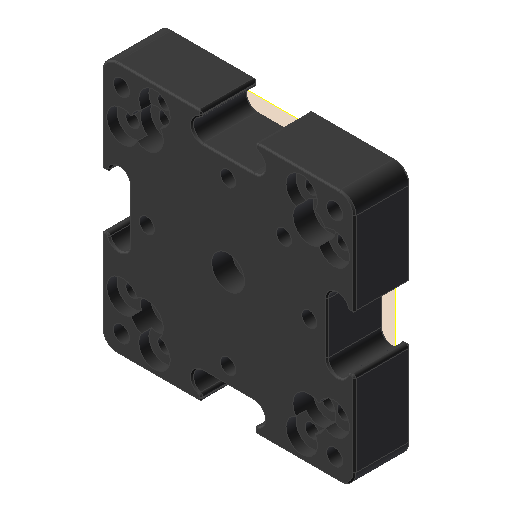
# Autodesk Inventor part: 40_XYZstage_micrometer_motorized_nema8_cube_ontop
Saved by Autodesk Inventor 2025.1 (Build 291241020, 241B)
## iProperties
Created: 2023-06-28
Part Number: 40_XYZstage_micrometer_motorized_nema8_cube_ontop
Material: Generisch
Document SubType Name: Modeling
Designer: diederichbenedict
Density: 1 g/cm^3
Appearance: Vorgabe
Author: diederichbenedict
Autodesk Inventor part; units mm, degrees
ref_plane "YZ Plane" through (0, 0, 0) normal (1, 0, 0) x (0, 1, 0)
ref_plane "XZ Plane" through (0, 0, 0) normal (0, 1, 0) x (-1, 0, 0)
ref_plane "XY Plane" through (0, 0, 0) normal (0, 0, 1) x (1, 0, 0)
ref_plane "Arbeitsebene1" through (0, 0, 0) normal (0, 0, 1) x (1, 0, 0)
sketch "Skizze1" plane through (0, 0, 0) normal (0, 0, 1) x (1, 0, 0)
  line L0 (0, -40) -> (0, 0) projected
  line L1 (0, 0) -> (-40, 0) projected
  line L2 (-40, 0) -> (-40, -40) projected
  line L3 (-40, -40) -> (0, -40) projected
  circle A0 centre (-20, -20) radius 1.5 projected
  circle A1 centre (-4, -20) radius 1.5 projected
  circle A2 centre (-4, -4) radius 1.5 projected
  circle A3 centre (-20, -4) radius 1.5 projected
  circle A4 centre (-36, -4) radius 1.5 projected
  circle A5 centre (-36, -20) radius 1.5 projected
  circle A6 centre (-36, -36) radius 1.5 projected
  circle A7 centre (-20, -36) radius 1.5 projected
  circle A8 centre (-4, -36) radius 1.5 projected
  circle A9 centre (-9, -8.5) radius 1.5 projected
  line L4 (1.9, 4.9) -> (-41.9, 4.9)
  line L5 (-44.9, 1.9) -> (-44.9, -41.9)
  line L6 (-41.9, -44.9) -> (1.9, -44.9)
  line L7 (4.9, -41.9) -> (4.9, 1.9)
  line L8 (4.9, 4.9) -> (-44.9, -44.9) construction
  line L9 (-44.9, 4.9) -> (4.9, -44.9) construction
  arc A10 (-44.9, -41.9) -> (-41.9, -44.9) centre (-41.9, -41.9) ccw
  arc A11 (-41.9, 4.9) -> (-44.9, 1.9) centre (-41.9, 1.9) ccw
  arc A12 (4.9, 1.9) -> (1.9, 4.9) centre (1.9, 1.9) ccw
  arc A13 (1.9, -44.9) -> (4.9, -41.9) centre (1.9, -41.9) ccw
  line L10 (1, 1) -> (-41, 1) construction
  line L11 (-41, 1) -> (-41, -41) construction
  line L12 (-41, -41) -> (1, -41) construction
  line L13 (1, -41) -> (1, 1) construction
  line L14 (1, 1) -> (-41, -41) construction
  line L15 (-41, 1) -> (1, -41) construction
  circle A14 centre (-41, -41) radius 1.6
  circle A15 centre (1, 1) radius 1.6
  circle A16 centre (1, -41) radius 1.6
  circle A17 centre (-41, 1) radius 1.6
  point P0 (-40, -0.249)
  point P1 (-39.751, 0)
  dimension "d0" = 49.8
  dimension "d1" = 49.8
  dimension "d2" = 3
  dimension "d3" = 42
  dimension "d4" = 42
  dimension "d5" = 3.2
  dimension "d7" = 3.2
  dimension "d8" = 3.2
  dimension "d33" = 3.2
  constraints: 24 end point, 8 centre point, 8 point on circle, 8 point on line, 8 tangent, 4 coincident, 4 midpoint, 4 parallel, 3 equal radius, 2 horizontal, 2 perpendicular
  measures "d0" distance of L9.end L8.end
  measures "d1" distance of L8.end L9.start
  measures "d2" radius of A10
  measures "d3" distance of L12.end L11.end
  measures "d4" distance of L11.end L10.end
  measures "d5" diameter of A14
  measures "d7" diameter of A15
  measures "d8" diameter of A16
  measures "d33" diameter of A17
extrude "Extrusion1" add sketch "Skizze1" along normal blind 11 contours A16 L3 A14 L2 A17 L1 A15 L0 | A17 L2 L1 | A12 L7 A13 L6 A10 L5 A11 L4 picked at (-39.8596, -0.0297)
sketch "Skizze2" plane through (0, 0, 0) normal (0, 0, -1) x (-1, 0, 0)
  circle A0 centre (-1, -41) radius 1.6 projected
  circle A1 centre (-1, 1) radius 1.6 projected
  circle A2 centre (41, -41) radius 1.6 projected
  line L0 (1.6191, -39.3087) -> (1.7742, -42.4226)
  line L1 (1.7742, -42.4226) -> (-0.8449, -44.1138)
  line L2 (-0.8449, -44.1138) -> (-3.6191, -42.6913)
  line L3 (-3.6191, -42.6913) -> (-3.7742, -39.5774)
  line L4 (-3.7742, -39.5774) -> (-1.1551, -37.8862)
  line L5 (-1.1551, -37.8862) -> (1.6191, -39.3087)
  line L6 (1.5708, -0.7638) -> (-1.2421, -2.1083)
  line L7 (-1.2421, -2.1083) -> (-3.8129, -0.3444)
  line L8 (-3.8129, -0.3444) -> (-3.5708, 2.7638)
  line L9 (-3.5708, 2.7638) -> (-0.7579, 4.1083)
  line L10 (-0.7579, 4.1083) -> (1.8129, 2.3444)
  line L11 (1.8129, 2.3444) -> (1.5708, -0.7638)
  line L12 (38.3642, -42.665) -> (38.2401, -39.5498)
  line L13 (38.2401, -39.5498) -> (40.8759, -37.8848)
  line L14 (40.8759, -37.8848) -> (43.6358, -39.335)
  line L15 (43.6358, -39.335) -> (43.7599, -42.4502)
  line L16 (43.7599, -42.4502) -> (41.1241, -44.1152)
  line L17 (41.1241, -44.1152) -> (38.3642, -42.665)
  line L18 (38.4992, -0.8617) -> (38.1373, 2.2349)
  line L19 (38.1373, 2.2349) -> (40.6381, 4.0966)
  line L20 (40.6381, 4.0966) -> (43.5008, 2.8617)
  line L21 (43.5008, 2.8617) -> (43.8627, -0.2349)
  line L22 (43.8627, -0.2349) -> (41.3619, -2.0966)
  line L23 (41.3619, -2.0966) -> (38.4992, -0.8617)
  arc A3 (40, -0.249) -> (39.751, 0) centre (41, 1) ccw projected
  point P0 (0, 0)
  dimension "d11" = 5.4
  dimension "d12" = 5.4
  dimension "d13" = 5.4
  dimension "d14" = 5.4
  constraints: 48 end point, 5 coincident, 52 other
  measures "d11" distance between parallel lines of L14 L17
  measures "d12" distance between parallel lines of L20 L23
  measures "d13" distance between parallel lines of L2 L5
  measures "d14" distance between parallel lines of L10 L7
extrude "Extrusion2" cut sketch "Skizze2" against normal blind 2.6 contours A0 | A1 | A2 | L0 L1 L2 L3 L4 L5 | L6 L7 L8 L9 L10 L11 | L12 L13 L14 L15 L16 L17 | L18 L19 L20 L21 L22 L23
sketch "Skizze3" plane through (0, 0, 11) normal (0, 0, 1) x (1, 0, 0)
  circle A0 centre (-36, -36) radius 1.5 projected
  circle A1 centre (-36, -4) radius 1.5 projected
  circle A2 centre (-4, -4) radius 1.5 projected
  circle A3 centre (-4, -36) radius 1.5 projected
  circle A4 centre (-20, -20) radius 1.5 projected
  point P0 (0, 0)
hole "Bohrung1" at (-36, -4, 11) at (-4, -4, 11) at (-4, -36, 11) at (-36, -36, 11) at (-20, -20, 11) direction (0, 0, -1) diameter 3.2 end through all counterbore diameter 6.5 counterbore depth 4
sketch "Skizze4" plane through (0, 0, 11) normal (0, 0, 1) x (1, 0, 0)
  arc A0 (-43.3711, -25.6646) -> (-39.55, -25.05) centre (-41.51, -25.05) ccw projected
  arc A1 (-43.3711, -25.6646) -> (-44.0833, -25.1498) centre (-44.0833, -25.8998) ccw projected
  line L0 (-44.0833, -25.1498) -> (-45, -25.1497) projected
  line L1 (-39.55, -14.95) -> (-39.55, -25.05) projected
  arc A2 (-39.55, -14.95) -> (-43.3711, -14.3354) centre (-41.51, -14.95) ccw projected
  arc A3 (-44.0833, -14.8502) -> (-43.3711, -14.3354) centre (-44.0833, -14.1002) ccw projected
  arc A4 (-45, -14.1002) -> (-44.2499, -14.8502) centre (-44.25, -14.1002) ccw projected
  line L2 (-44.2499, -14.8502) -> (-44.0833, -14.8502) projected
  line L3 (-45, -25.1497) -> (-45, -43) projected
  line L4 (-45, 3) -> (-45, -14.1002) projected
  line L5 (-45, -26) -> (-45, -14.1002)
  line L6 (-44.9, 1.9) -> (-44.9, -41.9) projected
  line L7 (-44.9, -43) -> (-44.9, -25.2497)
  line L8 (-44.9, -25.2497) -> (-44.0833, -25.2498)
  arc A5 (-43.4661, -25.6959) -> (-44.0833, -25.2498) centre (-44.0833, -25.8998) ccw
  arc A6 (-43.4661, -25.6959) -> (-39.45, -25.05) centre (-41.51, -25.05) ccw
  line L9 (-39.45, -25.05) -> (-39.45, -14.95)
  arc A7 (-39.45, -14.95) -> (-43.4661, -14.3041) centre (-41.51, -14.95) ccw
  arc A8 (-44.0833, -14.7502) -> (-43.4661, -14.3041) centre (-44.0833, -14.1002) ccw
  line L10 (-44.0833, -14.7502) -> (-44.2499, -14.7502)
  arc A9 (-44.9, -14.1002) -> (-44.2499, -14.7502) centre (-44.25, -14.1002) ccw
  line L11 (-44.9, -14.1002) -> (-44.9, 3)
  arc A10 (-44.25, -25.2498) -> (-45, -26) centre (-44.051, -26.1987) ccw
  point P0 (0, 0)
  point P1 (-44.9, -14.4744)
  dimension "d24" = 0.1
  constraints: 12 end point, 12 point on circle, 6 centre point, 2 point on line, 1 parallel, 9 other
  measures "d24" radial gap between concentric circles of A1 A5
extrude "Extrusion3" cut sketch "Skizze4" against normal through all
pattern_circular "Runde Anordnung1" count 4 over 360 about axis through (-20, -20, 0) along (0, 0, 1) of "Extrusion3"
chamfer "Fase1" distance 0.3 angle 45 88 edges at (-44.9, -33.8152, 11) (-44.0213, -44.0213, 11) (-33.8999, -44.9, 11) (-25.4401, -44.7096, 11) (-25.2498, -44.1666, 11) (-25.373, -43.7025, 11) (-27.0839, -41.1829, 11) (-20, -39.45, 11) (-12.9161, -41.1829, 11) (-14.627, -43.7025, 11) (-14.7502, -44.1666, 11) (-41.1829, -27.0839, 11) (-43.7025, -25.373, 11) (-44.1666, -25.2498, 11) (-39.45, -20, 11) (-41.1829, -12.9161, 11) (-43.7025, -14.627, 11) (-44.1666, -14.7502, 11) (-44.7096, -14.5599, 11) (-44.9, -6.1001, 11) (-44.0213, 4.0213, 11) (-33.8152, 4.9, 11) (-6.1848, -44.9, 11) (4.0213, -44.0213, 11) (4.9, -33.8999, 11) (4.7096, -25.4401, 11) (4.1666, -25.2498, 11) (3.7025, -25.373, 11) (1.1829, -27.0839, 11) (-0.55, -20, 11) (1.1829, -12.9161, 11) (3.7025, -14.627, 11) (4.1666, -14.7502, 11) (-12.9161, 1.1829, 11) (-20, -0.55, 11) (-27.0839, 1.1829, 11) (-25.373, 3.7025, 11) (-25.2498, 4.1666, 11) (-14.627, 3.7025, 11) (-14.7502, 4.1666, 11) (-14.5599, 4.7096, 11) (-6.1001, 4.9, 11) (4.0213, 4.0213, 11) (4.9, -6.1848, 11) (4.9, -33.8999, 0) (4.7096, -25.4401, 0) (4.1666, -25.2498, 0) (3.7025, -25.373, 0) (1.1829, -27.0839, 0) (-0.55, -20, 0) (1.1829, -12.9161, 0) (3.7025, -14.627, 0) (4.1666, -14.7502, 0) (4.0213, -44.0213, 0) (-6.1848, -44.9, 0) (4.9, -6.1848, 0) (4.0213, 4.0213, 0) (-6.1001, 4.9, 0) (-14.5599, 4.7096, 0) (-14.7502, 4.1666, 0) (-14.627, 3.7025, 0) (-12.9161, 1.1829, 0) (-20, -0.55, 0) (-27.0839, 1.1829, 0) (-25.373, 3.7025, 0) (-25.2498, 4.1666, 0) (-33.8152, 4.9, 0) (-44.9, -6.1001, 0) (-44.7096, -14.5599, 0) (-44.1666, -14.7502, 0) (-43.7025, -14.627, 0) (-41.1829, -12.9161, 0) (-39.45, -20, 0) (-41.1829, -27.0839, 0) (-43.7025, -25.373, 0) (-44.1666, -25.2498, 0) (-44.0213, 4.0213, 0) (-44.9, -33.8152, 0) (-44.0213, -44.0213, 0) (-33.8999, -44.9, 0) (-25.4401, -44.7096, 0) (-25.2498, -44.1666, 0) (-25.373, -43.7025, 0) (-27.0839, -41.1829, 0) (-20, -39.45, 0) (-12.9161, -41.1829, 0) (-14.627, -43.7025, 0) (-14.7502, -44.1666, 0)
sketch "Sketch6" plane through (0, 0, 11) normal (0, 0, 1) x (1, 0, 0)
  circle A0 centre (1, 1) radius 1.6 projected
  circle A1 centre (-4, -20) radius 1.5 projected
  circle A2 centre (-20, -4) radius 1.5 projected
  circle A3 centre (-36, -20) radius 1.5 projected
  circle A4 centre (-20, -36) radius 1.5 projected
  circle A5 centre (-9, -8.5) radius 1.5 projected
  circle A6 centre (1, -41) radius 1.6 projected
  circle A7 centre (-41, -41) radius 1.6 projected
  arc A8 (-39.751, 0) -> (-40, -0.249) centre (-41, 1) ccw projected
  line L0 (-39.751, 0) -> (-40, 0) projected
  line L1 (-40, 0) -> (-40, -0.249) projected
  circle A9 centre (-20, -20) radius 3.25 projected
  circle A10 centre (-4, -36) radius 3.25 projected
  circle A11 centre (-36, -4) radius 3.25 projected
  circle A12 centre (-4, -4) radius 3.25 projected
  circle A13 centre (-36, -36) radius 3.25 projected
  line L2 (4.6, 1.9) -> (4.6, -14.4503) projected
  arc A14 (4.6, 1.9) -> (1.9, 4.6) centre (1.9, 1.9) ccw projected
  line L3 (-14.1002, 4.6) -> (1.9, 4.6) projected
  arc A15 (-14.1002, 4.6) -> (-14.4502, 4.25) centre (-14.1002, 4.25) ccw projected
  line L4 (-14.4502, 4.0833) -> (-14.4502, 4.25) projected
  arc A16 (-14.4502, 4.0833) -> (-14.21, 3.751) centre (-14.1002, 4.0833) ccw projected
  arc A17 (-14.95, -0.85) -> (-14.21, 3.751) centre (-14.95, 1.51) ccw projected
  line L5 (-25.05, -0.85) -> (-14.95, -0.85) projected
  arc A18 (-25.79, 3.751) -> (-25.05, -0.85) centre (-25.05, 1.51) ccw projected
  arc A19 (-25.79, 3.751) -> (-25.5498, 4.0833) centre (-25.8998, 4.0833) ccw projected
  line L6 (-25.5497, 4.6) -> (-25.5498, 4.0833) projected
  line L7 (-41.9, 4.6) -> (-25.5497, 4.6) projected
  arc A20 (-41.9, 4.6) -> (-44.6, 1.9) centre (-41.9, 1.9) ccw projected
  line L8 (-44.6, -14.1002) -> (-44.6, 1.9) projected
  arc A21 (-44.6, -14.1002) -> (-44.25, -14.4502) centre (-44.25, -14.1002) ccw projected
  line L9 (-44.0833, -14.4502) -> (-44.25, -14.4502) projected
  arc A22 (-44.0833, -14.4502) -> (-43.751, -14.21) centre (-44.0833, -14.1002) ccw projected
  arc A23 (-39.15, -14.95) -> (-43.751, -14.21) centre (-41.51, -14.95) ccw projected
  line L10 (-39.15, -25.05) -> (-39.15, -14.95) projected
  arc A24 (-43.751, -25.79) -> (-39.15, -25.05) centre (-41.51, -25.05) ccw projected
  arc A25 (-43.751, -25.79) -> (-44.0833, -25.5498) centre (-44.0833, -25.8998) ccw projected
  line L11 (-44.6, -25.5497) -> (-44.0833, -25.5498) projected
  line L12 (-44.6, -41.9) -> (-44.6, -25.5497) projected
  arc A26 (-44.6, -41.9) -> (-41.9, -44.6) centre (-41.9, -41.9) ccw projected
  line L13 (-25.8998, -44.6) -> (-41.9, -44.6) projected
  arc A27 (-25.8998, -44.6) -> (-25.5498, -44.25) centre (-25.8998, -44.25) ccw projected
  line L14 (-25.5498, -44.0833) -> (-25.5498, -44.25) projected
  arc A28 (-25.5498, -44.0833) -> (-25.79, -43.751) centre (-25.8998, -44.0833) ccw projected
  arc A29 (-25.05, -39.15) -> (-25.79, -43.751) centre (-25.05, -41.51) ccw projected
  line L15 (-14.95, -39.15) -> (-25.05, -39.15) projected
  arc A30 (-14.21, -43.751) -> (-14.95, -39.15) centre (-14.95, -41.51) ccw projected
  arc A31 (-14.21, -43.751) -> (-14.4502, -44.0833) centre (-14.1002, -44.0833) ccw projected
  line L16 (-14.4503, -44.6) -> (-14.4502, -44.0833) projected
  line L17 (1.9, -44.6) -> (-14.4503, -44.6) projected
  arc A32 (1.9, -44.6) -> (4.6, -41.9) centre (1.9, -41.9) ccw projected
  line L18 (4.6, -25.8998) -> (4.6, -41.9) projected
  arc A33 (4.6, -25.8998) -> (4.25, -25.5498) centre (4.25, -25.8998) ccw projected
  line L19 (4.0833, -25.5498) -> (4.25, -25.5498) projected
  arc A34 (4.0833, -25.5498) -> (3.751, -25.79) centre (4.0833, -25.8998) ccw projected
  arc A35 (-0.85, -25.05) -> (3.751, -25.79) centre (1.51, -25.05) ccw projected
  line L20 (-0.85, -14.95) -> (-0.85, -25.05) projected
  arc A36 (3.751, -14.21) -> (-0.85, -14.95) centre (1.51, -14.95) ccw projected
  arc A37 (3.751, -14.21) -> (4.0833, -14.4502) centre (4.0833, -14.1002) ccw projected
  line L21 (4.6, -14.4503) -> (4.0833, -14.4502) projected
  line L22 (-40.8, -34.5) -> (-40.8, -5.5)
  line L23 (-40.8, -5.5) -> (0.8, -5.5)
  line L24 (0.8, -5.5) -> (0.8, -34.5)
  line L25 (0.8, -34.5) -> (-40.8, -34.5)
  line L26 (-40.8, -34.5) -> (0.8, -5.5) construction
  line L27 (-40.8, -5.5) -> (0.8, -34.5) construction
  line L28 (-40.8, -34.5) -> (-11.8, -34.5) construction
  line L29 (-34.5, -40.75) -> (-34.5, 0.75)
  line L30 (-34.5, 0.75) -> (-5.5, 0.75)
  line L31 (-5.5, 0.75) -> (-5.5, -40.75)
  line L32 (-5.5, -40.75) -> (-34.5, -40.75)
  line L33 (-34.5, -40.75) -> (-5.5, 0.75) construction
  line L34 (-34.5, 0.75) -> (-5.5, -40.75) construction
  line L35 (1.9, 4.9) -> (-14.1002, 4.9) projected
  line L36 (-34.5, -40.75) -> (7, -40.75) construction
  point P0 (0, 0)
  dimension "d39" = 29
  dimension "d40" = 90
  dimension "d41" = 41.6
  dimension "d42" = 41.5
  dimension "d43" = 90
  dimension "d44" = 29
  constraints: 28 end point, 5 perpendicular, 4 midpoint, 4 parallel, 2 horizontal, 1 vertical
  measures "d39" distance of L22.start L22.end
  measures "d40" angle of L28 L22
  measures "d41" distance of L22.end L23.end
  measures "d42" distance of L29.start L29.end
  measures "d43" angle of L36 L29
  measures "d44" distance of L29.end L30.end
hole "Hole2" at (-34.5, 0.75, 11) at (-40.8, -5.5, 11) at (-40.8, -34.5, 11) at (-34.5, -40.75, 11) at (-5.5, -40.75, 11) at (0.8, -34.5, 11) at (0.8, -5.5, 11) at (-5.5, 0.75, 11) direction (0, 0, -1) diameter 2.7 end through all counterbore diameter 6.2 counterbore depth 2
equation "\"d12\" = d11"
equation "\"d13\" = d11"
equation "\"d14\" = d11"
